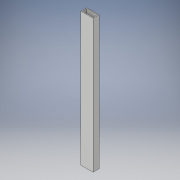
# Autodesk Inventor part: ElectricalBoardSupport.ver1-1111-2019
Saved by Autodesk Inventor 2018 (Build 220112000, 112)
## iProperties
Created: 2019-11-12
Part Number: ElectricalBoardSupport.ver1-1111-2019
Material: Generic
Document SubType Name: Modeling
Designer: JMHal
Density: 1 g/cm^3
Appearance: Default
Author: JMHal
Autodesk Inventor part; units mm, degrees
ref_plane "YZ Plane" through (0, 0, 0) normal (1, 0, 0) x (0, 1, 0)
ref_plane "XZ Plane" through (0, 0, 0) normal (0, 1, 0) x (-1, 0, 0)
ref_plane "XY Plane" through (0, 0, 0) normal (0, 0, 1) x (1, 0, 0)
sketch "Sketch1" plane through (0, 0, 0) normal (0, 1, 0) x (-1, 0, 0)
  line L0 (0, 0) -> (50.8, 0)
  line L1 (50.8, 0) -> (50.8, -25.4)
  line L2 (50.8, -25.4) -> (0, -25.4)
  line L3 (0, -25.4) -> (0, 0)
  line L4 (47.625, -22.225) -> (47.625, -3.175)
  line L5 (47.625, -3.175) -> (3.175, -3.175)
  line L6 (3.175, -3.175) -> (3.175, -22.225)
  line L7 (3.175, -22.225) -> (47.625, -22.225)
  dimension "d0" = 50.8
  dimension "d1" = 25.4
  dimension "d2" = 3.175
  constraints: 16 end point, 4 parallel, 2 perpendicular, 1 horizontal, 3 other
  measures "d0" distance of L1.end L2.end
  measures "d1" distance of L0.end L1.end
  measures "d2" distance between parallel lines of L1 L4
extrude "Extrusion1" add sketch "Sketch1" along normal blind 584.2
sketch "Sketch2" plane through (0, 584.2, 0) normal (0, 1, 0) x (1, 0, 0)
  line L0 (-47.625, 22.225) -> (-3.175, 22.225) projected
  line L1 (-3.175, 22.225) -> (-3.175, 3.175) projected
  line L2 (-3.175, 3.175) -> (-47.625, 3.175) projected
  line L3 (-47.625, 3.175) -> (-47.625, 22.225) projected
  line L4 (-50.8, 0) -> (0, 0) projected
  line L5 (0, 0) -> (0, 25.4) projected
  line L6 (0, 25.4) -> (-50.8, 25.4) projected
  line L7 (-50.8, 25.4) -> (-50.8, 0) projected
extrude "Extrusion2" cut sketch "Sketch2" against normal blind 25.4
body "Solid1"
